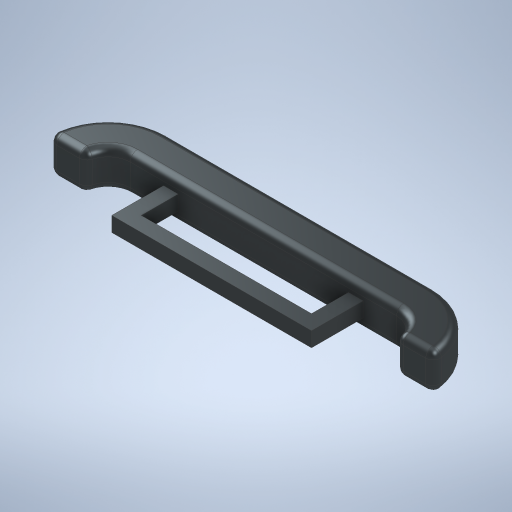
# Autodesk Inventor part: bumper
Saved by Autodesk Inventor 2023 (Build 270158000, 158)
## iProperties
Created: 2024-02-05
Part Number: bumper
Material: 일반
Document SubType Name: Modeling
Designer: ps737
Density: 1 g/cm^3
Appearance: 기본값
Author: ps737
Autodesk Inventor part; units mm, degrees
ref_plane "YZ Plane" through (0, 0, 0) normal (1, 0, 0) x (0, 1, 0)
ref_plane "XZ Plane" through (0, 0, 0) normal (0, 1, 0) x (-1, 0, 0)
ref_plane "XY Plane" through (0, 0, 0) normal (0, 0, 1) x (1, 0, 0)
sketch "스케치1" plane through (0, 0, 0) normal (0, 1, 0) x (-1, 0, 0)
  line L0 (270, 0) -> (-270, 0)
  line L1 (270, 0) -> (270, -240)
  line L2 (270, -240) -> (230, -240)
  line L3 (230, -240) -> (230, -40)
  line L4 (230, -40) -> (-230, -40)
  line L5 (-230, -40) -> (-230, -240)
  line L6 (-230, -240) -> (-270, -240)
  line L7 (-270, -240) -> (-270, 0)
  line L8 (-560, -240) -> (480, -240)
  arc A0 (360, -240) -> (520, -80) centre (360, -80) ccw
  arc A1 (360, -140) -> (420, -80) centre (360, -80) ccw
  line L9 (420, -80) -> (520, -80)
  line L10 (360, -140) -> (-40, -140)
  arc A2 (-520, -80) -> (-360, -240) centre (-360, -80) ccw
  arc A3 (-420, -80) -> (-360, -140) centre (-360, -80) ccw
  line L11 (-420, -80) -> (-520, -80)
  line L12 (-360, -140) -> (-40, -140)
  line L13 (360, -240) -> (-360, -240)
  point P0 (0, 0)
  point P1 (0, 0)
  point P2 (-270, -140)
  point P3 (-230, -140)
  point P4 (230, -140)
  point P5 (270, -140)
  dimension "d1" = 240
  dimension "d2" = 40
  dimension "d3" = 200
  dimension "d4" = 460
  dimension "d6" = 1040
  dimension "d9" = 240
  dimension "d11" = 100
  dimension "d12" = 160
  dimension "d13" = 160
  dimension "d14" = 160
  dimension "d17" = 210
  dimension "d18" = 310
  dimension "d24" = 270
  dimension "d25" = 0
  dimension "d26" = 250
  dimension "d27" = 60
  dimension "d28" = 0
  dimension "d29" = 160
  dimension "d30" = 0
  dimension "d31" = 60
  dimension "d32" = 40
  dimension "d33" = 160
  dimension "d34" = 40
  dimension "d35" = 60
  dimension "d36" = 500
  dimension "d37" = 160
  dimension "d38" = 500
  dimension "d39" = 60
  dimension "d40" = 540
  dimension "d41" = 160
  dimension "d42" = 540
  dimension "d43" = 630
  dimension "d44" = 160
  dimension "d45" = 630
  constraints: 28 end point, 8 point on circle, 5 perpendicular, 4 centre point, 4 tangent, 3 horizontal, 3 parallel, 1 coincident, 1 collinear, 1 equal radius, 1 midpoint, 1 point on line, 1 vertical
  measures "d1" distance of L0.start L1.end
  measures "d2" distance of L1.end L2.end
  measures "d3" distance of L2.end L3.end
  measures "d4" distance of L3.end L4.end
  measures "d6" distance of L8.start L8.end
  measures "d9" distance between parallel lines of L0 L8
  measures "d11" radial gap between concentric circles of A0 A1
  measures "d12" radius of A0
  measures "d13" distance between parallel lines of L9 L2
  measures "d14" distance between parallel lines of L9 L6
  measures "d17" distance from line of L8.end L1
  measures "d18" distance from line of L10.end L1
  measures "d24" distance from line of L1 point (0, 0)
  measures "d25" distance between parallel lines of L9 L11
  measures "d26" distance from line of L9.end L1
  measures "d27" distance from line of point (270, -140) L9
  measures "d28" distance from line of point (270, -140) L1
  measures "d29" distance from line of point (270, -240) L9
  measures "d30" distance from line of point (270, -240) L1
  measures "d31" distance from line of point (230, -140) L9
  measures "d32" distance from line of point (230, -140) L1
  measures "d33" distance from line of point (230, -240) L9
  measures "d34" distance from line of point (230, -240) L1
  measures "d35" distance from line of point (-230, -140) L9
  measures "d36" distance from line of point (-230, -140) L1
  measures "d37" distance from line of point (-230, -240) L9
  measures "d38" distance from line of point (-230, -240) L1
  measures "d39" distance from line of point (-270, -140) L9
  measures "d40" distance from line of point (-270, -140) L1
  measures "d41" distance from line of point (-270, -240) L9
  measures "d42" distance from line of point (-270, -240) L1
  measures "d43" distance from line of A3.centre L1
  measures "d44" distance from line of point (-360, -240) L9
  measures "d45" distance from line of point (-360, -240) L1
extrude "돌출3" add sketch "스케치1" along normal mid plane 40 contours L1 L10 L3 L4 L5 L12 L7 L0
extrude "돌출4" add sketch "스케치1" along normal mid plane 100 contours L10 A1 L9 A0 L8 L1 | L1 L2 L3 L10 | L12 L5 L6 L7 | L7 L8 A2 L11 A3 L12 | L3 L8 L5 L12 L10
fillet "모깎기1" radius 20 20 edges at (-473.1371, 50, -193.1371) (473.1371, 50, -193.1371) (0, 50, -240) (0, -50, -240) (-473.1371, -50, -193.1371) (473.1371, -50, -193.1371) (470, 50, -80) (402.4264, 50, -122.4264) (-402.4264, 50, -122.4264) (0, 50, -140) (470, -50, -80) (-402.4264, -50, -122.4264) (402.4264, -50, -122.4264) (0, -50, -140) (-470, -50, -80) (-470, 50, -80) (-520, 0, -80) (-420, 0, -80) (420, 0, -80) (520, 0, -80)
